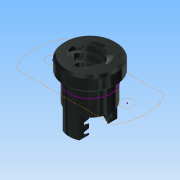
# Autodesk Inventor part: screw t8
Saved by Autodesk Inventor 2017 (Build 210142000, 142)
## iProperties
Part Number: screw t8
Material: Типовые
Document SubType Name: Modeling
Designer: alcapone
Density: 1 g/cm^3
Appearance: Оружейный металл — полированный
Mass: 0.587825 g
Surface Area: 10.6675 cm^2
Volume: 0.587825 cm^3
Author: alcapone
Autodesk Inventor part; units mm, degrees
ref_plane "YZ Plane" through (0, 0, 0) normal (1, 0, 0) x (0, 1, 0)
ref_plane "XZ Plane" through (0, 0, 0) normal (0, 1, 0) x (-1, 0, 0)
ref_plane "XY Plane" through (0, 0, 0) normal (0, 0, 1) x (1, 0, 0)
sketch "Эскиз6" plane through (0, 0, 0) normal (0, 0, 1) x (1, 0, 0)
  arc A0 (11.7132, -6.3) -> (11.7132, 6.3) centre (1.5, 0) ccw construction
  line L0 (11.7132, 6.3) -> (-11.7132, 6.3) construction
  arc A1 (-11.7132, 6.3) -> (-11.7132, -6.3) centre (-1.5, 0) ccw construction
  line L1 (-11.7132, -6.3) -> (11.7132, -6.3) construction
  circle A2 centre (-9, 0) radius 1.5 construction
  circle A3 centre (9, 0) radius 1.5 construction
  circle A4 centre (0, 0) radius 5
  circle A5 centre (0, 0) radius 5
  circle A6 centre (0, 0) radius 4
  circle A7 centre (0, 0) radius 3
  dimension "d23" = 6
  constraints: 8 centre point, 4 end point, 4 point on circle, 1 coincident
  measures "d23" diameter of A7
extrude "Выдавливание5" add sketch "Эскиз6" against normal blind 9 contours A4 | A6
extrude "Выдавливание6" add sketch "Эскиз6" along normal blind 5.5 contours A4 | A6
sketch "Эскиз2" plane through (0, 0, 0) normal (0, 0, 1) x (1, 0, 0)
  circle A0 centre (0, 0) radius 4
  dimension "d0" = 8
  constraints: 1 centre point, 1 coincident
  measures "d0" diameter of A0
sketch "Эскиз7" plane through (0, 0, 0) normal (0, 1, 0) x (-1, 0, 0)
  line L0 (0, -13.5272) -> (0, 21.8679) construction
  line L1 (0, -13.5272) -> (5.4466, -13.5272) construction
  line L2 (4, -13.5272) -> (3, -13.5272)
  line L3 (3, -13.5272) -> (3, -12.5272)
  line L4 (3, -12.5272) -> (4, -12.5272)
  line L5 (4, -12.5272) -> (4, -13.5272)
  point P0 (0, 0)
  dimension "d30" = 1
  dimension "d31" = 1
  dimension "d32" = 3
  constraints: 12 end point, 2 horizontal, 2 parallel, 1 perpendicular, 1 point on line, 1 vertical
  measures "d30" distance between parallel lines of L1 L4
  measures "d31" distance between parallel lines of L3 L5
  measures "d32" distance between parallel lines of L0 L3
coil "Пружина2" sketch "Эскиз7" operation cut axis through (0, 0, -13.5272) along (0, 0, 1) pitch 8 turns 4 hand right
pattern_circular "Круговой массив2" count 4 over 360 about axis through (0, 0, 0) along (0, 0, -1) of "Пружина2"
sketch "Эскиз10" plane through (0, 0, 5.5) normal (0, 0, 1) x (1, 0, 0)
  circle A0 centre (0, 0) radius 6.3
  circle A1 centre (0, 0) radius 5
  dimension "d54" = 12.6
  constraints: 2 centre point, 2 coincident
  measures "d54" diameter of A0
extrude "Выдавливание8" add sketch "Эскиз10" against normal blind 3.5
chamfer "Фаска3" distance 0.5 angle 45 2 edges at (-6.3, 0, 5.5) (-6.3, 0, 2)
sketch "Эскиз11" plane through (0, 0, 0) normal (0, 1, 0) x (-1, 0, 0)
  line L0 (2, -12.7493) -> (-2, -12.7493)
  line L1 (-2, -12.7493) -> (-2, -4)
  line L2 (-2, -4) -> (2, -4)
  line L3 (2, -4) -> (2, -12.7493)
  line L4 (0, 0) -> (0, -18.4973) construction
  line L5 (2, -4) -> (6.456, -4)
  line L6 (6.456, -4) -> (6.456, -12.7493)
  line L7 (6.456, -12.7493) -> (2, -12.7493)
  line L8 (2, -12.7493) -> (2, -4)
  line L9 (-2, -4) -> (-8.056, -4)
  line L10 (-8.056, -4) -> (-8.056, -12.7493)
  line L11 (-8.056, -12.7493) -> (-2, -12.7493)
  line L12 (-2, -12.7493) -> (-2, -4)
  line L13 (2.7955, -9) -> (1.207, -9) projected
  dimension "d60" = 5
  dimension "d61" = 4
  constraints: 26 end point, 6 parallel, 3 horizontal, 3 perpendicular, 1 point on line, 1 vertical, 1 other
  measures "d60" distance between parallel lines of L13 L2
  measures "d61" distance between parallel lines of L1 L3
extrude "Выдавливание9" cut sketch "Эскиз11" along normal mid plane 20 contours L3 L5 L6 L7 | L11 L10 L9 L1
